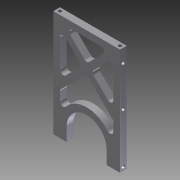
# Autodesk Inventor part: lower box front plate2
Saved by Autodesk Inventor 2012 (Build 160160000, 160)
## iProperties
Created: 2012-07-05
Part Number: lower box front plate2
Material: Default
Document SubType Name: Modeling
Designer: Bryce
Density: 1 g/cm^3
Author: Bryce
Autodesk Inventor part; units mm, degrees
ref_plane "YZ Plane" through (0, 0, 0) normal (1, 0, 0) x (0, 1, 0)
ref_plane "XZ Plane" through (0, 0, 0) normal (0, 1, 0) x (-1, 0, 0)
sketch "Sketch1" plane through (0, 0, 0) normal (0, 0, 1) x (1, 0, 0)
  line L0 (-31.75, 110.3249) -> (31.75, 110.3249)
  line L1 (31.75, 110.3249) -> (31.75, 8.7249)
  line L2 (-31.75, 8.7249) -> (-31.75, 110.3249)
  line L3 (-31.75, 8.7249) -> (-19.05, 8.7249)
  line L4 (31.75, 8.7249) -> (19.05, 8.7249)
  line L5 (-19.05, 8.7249) -> (-19.05, 21.4249)
  line L6 (19.05, 8.7249) -> (19.05, 21.4249)
  arc A0 (19.05, 21.4249) -> (-19.05, 21.4249) centre (0, 21.4249) ccw
  point P0 (0, 0)
  dimension "d0" = 63.5
  dimension "d1" = 31.75
  dimension "d2" = 101.6
  dimension "d3" = 110.3249
  dimension "d4" = 12.7
  dimension "d5" = 12.7
  dimension "d46" = 101.6
  dimension "d52" = 12.7
  dimension "d53" = 12.7
  constraints: 14 end point, 3 equal length, 3 perpendicular, 2 point on circle, 1 centre point, 1 horizontal, 1 tangent
  measures "d0" distance of L0.start L0.end
  measures "d1" distance from line of L1 point (0, 0)
  measures "d2" distance of L0.end L1.end
  measures "d3" distance from line of L0 point (0, 0)
  measures "d4" distance of L2.start L3.end
  measures "d5" distance of L1.end L4.end
  measures "d46" distance of L2.start L0.start
  measures "d52" distance of L3.end L5.end
  measures "d53" distance of L4.end L6.end
extrude "Extrusion1" add sketch "Sketch1" against normal blind 6.35
sketch "Sketch2" plane through (31.75, 8.7249, 0) normal (1, 0, 0) x (0, 0, -1)
  line L0 (6.35, 0) -> (6.35, 101.6) projected
  line L1 (0, 101.6) -> (6.35, 101.6) projected
  line L2 (0, 101.6) -> (0, 0) projected
  line L3 (0, 0) -> (6.35, 0) projected
  point P0 (0, -8.7249)
  point P1 (3.175, 3.175)
  point P2 (3.175, 88.9)
  point P3 (3.175, 50.8)
  dimension "d22" = 12.7
  dimension "d23" = 3.175
  dimension "d24" = 3.175
  dimension "d25" = 3.175
  dimension "d54" = 50.8
  dimension "d55" = 3.175
  measures "d22" distance from line of L1 point (3.175, 88.9)
  measures "d23" distance from line of L2 point (3.175, 88.9)
  measures "d24" distance from line of L3 point (3.175, 3.175)
  measures "d25" distance from line of L0 point (3.175, 3.175)
  measures "d54" distance from line of L3 point (3.175, 50.8)
  measures "d55" distance from line of L0 point (3.175, 50.8)
hole "Hole2" at (31.75, 11.8999, -3.175) at (31.75, 97.6249, -3.175) at (31.75, 59.5249, -3.175) direction (-1, 0, 0) diameter 3.175 depth 9.525 tip angle 118
sketch "Sketch3" plane through (-31.75, 8.7249, 0) normal (-1, 0, 0) x (0, 0, 1)
  line L0 (0, 0) -> (-6.35, 0) projected
  line L1 (0, 0) -> (0, 101.6) projected
  line L2 (0, 101.6) -> (-6.35, 101.6) projected
  line L3 (-6.35, 101.6) -> (-6.35, 0) projected
  point P0 (0, -8.7249)
  point P1 (-3.175, 88.9)
  point P2 (-3.175, 3.175)
  point P3 (-3.175, 50.8)
  dimension "d33" = 3.175
  dimension "d34" = 12.7
  dimension "d35" = 3.175
  dimension "d36" = 3.175
  dimension "d56" = 50.8
  dimension "d57" = 3.175
  measures "d33" distance from line of L1 point (-3.175, 88.9)
  measures "d34" distance from line of L2 point (-3.175, 88.9)
  measures "d35" distance from line of L0 point (-3.175, 3.175)
  measures "d36" distance from line of L1 point (-3.175, 3.175)
  measures "d56" distance from line of L0 point (-3.175, 50.8)
  measures "d57" distance from line of L3 point (-3.175, 50.8)
hole "Hole3" at (-31.75, 97.6249, -3.175) at (-31.75, 11.8999, -3.175) at (-31.75, 59.5249, -3.175) direction (1, 0, 0) diameter 3.175 depth 9.525 tip angle 118
sketch "Sketch5" plane through (-31.75, 110.3249, 0) normal (0, 1, 0) x (1, 0, 0)
  line L0 (0, 0) -> (0, 6.35) projected
  line L1 (0, 0) -> (63.5, 0) projected
  line L2 (63.5, 0) -> (63.5, 6.35) projected
  point P0 (31.75, 0)
  point P1 (3.175, 3.175)
  point P2 (60.325, 3.175)
  dimension "d78" = 3.175
  dimension "d79" = 3.175
  dimension "d80" = 3.175
  constraints: 1 horizontal alignment
  measures "d78" distance from line of L1 point (3.175, 3.175)
  measures "d79" distance from line of L0 point (3.175, 3.175)
  measures "d80" distance from line of L2 point (60.325, 3.175)
hole "Hole4" at (-28.575, 110.3249, -3.175) at (28.575, 110.3249, -3.175) direction (0, -1, 0) diameter 3.175 depth 9.525 tip angle 118
ref_plane "Work Plane2" through (0, 0, -3.175) normal (0, 0, 1) x (1, 0, 0)
sketch "Sketch6" plane through (0, 0, -3.175) normal (0, 0, 1) x (1, 0, 0)
  arc A0 (25.4, 21.4249) -> (-25.4, 21.4249) centre (0, 21.4249) ccw
  line L0 (-31.75, 110.3249) -> (-31.75, 8.7249) projected
  line L1 (31.75, 110.3249) -> (-31.75, 110.3249) projected
  line L2 (31.75, 8.7249) -> (31.75, 110.3249) projected
  line L3 (19.05, 8.7249) -> (31.75, 8.7249) projected
  arc A1 (19.05, 21.4249) -> (-19.05, 21.4249) centre (0, 21.4249) ccw projected
  line L4 (19.05, 21.4249) -> (19.05, 8.7249) projected
  line L5 (-19.05, 8.7249) -> (-19.05, 21.4249) projected
  line L6 (-31.75, 8.7249) -> (-19.05, 8.7249) projected
  line L7 (-25.4, 21.4249) -> (-25.4, 103.9749)
  line L8 (-25.4, 103.9749) -> (25.4, 103.9749)
  line L9 (25.4, 103.9749) -> (25.4, 21.4249)
  line L10 (25.4, 103.9749) -> (-25.4, 53.1749) construction
  line L11 (-25.4, 103.9749) -> (25.4, 53.1749) construction
  line L12 (-25.4, 99.4848) -> (-4.4901, 78.5749)
  line L13 (-4.4901, 78.5749) -> (-25.4, 57.665)
  line L14 (-20.9099, 103.9749) -> (0, 83.065)
  line L15 (0, 83.065) -> (20.9099, 103.9749)
  line L16 (25.4, 99.4848) -> (4.4901, 78.5749)
  line L17 (4.4901, 78.5749) -> (25.4, 57.665)
  line L18 (-25.4, 48.6848) -> (0, 74.0848)
  line L19 (0, 74.0848) -> (25.4, 48.6848)
  arc A2 (-25.4, 65.3302) -> (-19.9799, 63.0851) centre (-22.225, 65.3302) ccw
  arc A3 (-19.9799, 94.0647) -> (-25.4, 91.8196) centre (-22.225, 91.8196) ccw
  arc A4 (25.4, 91.8196) -> (19.9799, 94.0647) centre (22.225, 91.8196) ccw
  arc A5 (19.9799, 63.0851) -> (25.4, 65.3302) centre (22.225, 65.3302) ccw
  point P0 (0, 0)
  dimension "d99" = 25.4
  dimension "d100" = 6.35
  dimension "d101" = 6.35
  dimension "d102" = 6.35
  dimension "d103" = 45
  dimension "d104" = 6.35
  dimension "d105" = 3.175
  dimension "d106" = 3.175
  dimension "d108" = 6.35
  dimension "d109" = 3.175
  dimension "d110" = 6.35
  dimension "d111" = 3.175
  dimension "d112" = 6.35
  dimension "d113" = 3.175
  dimension "d114" = 3.175
  dimension "d115" = 3.175
  dimension "d116" = 3.175
  constraints: 26 end point, 18 point on line, 10 point on circle, 9 perpendicular, 8 tangent, 5 centre point, 4 parallel, 1 concentric
  measures "d99" radius of A0
  measures "d100" distance between parallel lines of L0 L7
  measures "d101" distance between parallel lines of L2 L9
  measures "d102" distance between parallel lines of L1 L8
  measures "d103" angle of L10 L8
  measures "d104" distance between parallel lines of L12 L14
  measures "d105" distance between parallel lines of L14 L11
  measures "d106" distance between parallel lines of L10 L15
  measures "d108" distance between parallel lines of L16 L15
  measures "d109" distance between parallel lines of L11 L17
  measures "d110" distance between parallel lines of L19 L17
  measures "d111" distance between parallel lines of L13 L10
  measures "d112" distance between parallel lines of L13 L18
  measures "d113" radius of A2
  measures "d114" radius of A3
  measures "d115" radius of A4
  measures "d116" radius of A5
extrude "Extrusion5" cut sketch "Sketch6" along normal mid plane 25.4 contours A0 L7 L18 L19 L9 | A5 L17 L16 A4 L9 | L7 A3 L12 L13 A2 | L15 L14 L8
fillet "Fillet3" radius 3.175 10 edges at (-25.4, 21.4249, -3.175) (25.4, 21.4249, -3.175) (25.4, 48.6848, -3.175) (0, 74.0848, -3.175) (-25.4, 48.6848, -3.175) (-4.4901, 78.5749, -3.175) (4.4901, 78.5749, -3.175) (0, 83.065, -3.175) (-20.9099, 103.9749, -3.175) (20.9099, 103.9749, -3.175)
equation "\"d105\" = 0.5 * d104"
equation "\"d106\" = d105"
equation "\"d109\" = d105"
equation "\"d110\" = d108"
equation "\"d111\" = d105"
equation "\"d112\" = d104"
body "Solid1"
